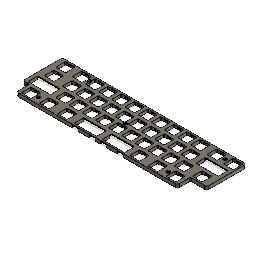
plate (Autodesk Fusion 360 design; units mm, degrees)
Autodesk Fusion 360 part; units mm, degrees
(part 1 of 9)
sketch "Sketch1" plane through (0, 0, 0) normal (0, 1, 0) x (1, 0, 0)
  line L0 (3, 0) -> (263.7, 0)
  line L1 (266.7, -3) -> (266.7, -73.2)
  line L2 (263.7, -76.2) -> (3, -76.2)
  line L3 (0, -73.2) -> (0, -3)
  arc A0 (3, 0) -> (0, -3) centre (3, -3) ccw
  arc A1 (0, -73.2) -> (3, -76.2) centre (3, -73.2) ccw
  arc A2 (266.7, -3) -> (263.7, 0) centre (263.7, -3) ccw
  arc A3 (263.7, -76.2) -> (266.7, -73.2) centre (263.7, -73.2) ccw
  point P0 (266.7, 0)
  point P1 (0, -76.2)
  dimension "d1" = 266.7
  dimension "d2" = 76.2
  dimension "d3" = 3
  constraint horizontal L0
  constraint vertical L1
  constraint horizontal L2
  constraint vertical L3
  constraint coincident origin L0
  constraint coincident origin L3
  constraint tangent L0 A0
  constraint tangent L3 A0
  constraint coincident P1 L2
  constraint coincident P1 L3
  constraint tangent L2 A1
  constraint tangent L3 A1
  constraint equal A0 A1
  constraint coincident P0 L0
  constraint coincident P0 L1
  constraint tangent L0 A2
  constraint tangent L1 A2
  constraint equal A0 A2
  constraint tangent L1 A3
  constraint tangent L2 A3
  constraint equal A0 A3
  measures "d1" distance of origin P0
  measures "d2" distance of origin P1
  measures "d3" radius of A0
extrude "Extrude1" add sketch "Sketch1" along normal blind 5.1
sketch "Sketch2" plane through (0, 5.1, 0) normal (0, 1, 0) x (-1, 0, 0)
  arc A0 (0, 73.2) -> (-3, 76.2) centre (-3, 73.2) ccw
  line L0 (-3, 76.2) -> (-263.7, 76.2)
  arc A1 (-263.7, 76.2) -> (-266.7, 73.2) centre (-263.7, 73.2) ccw
  line L1 (-266.7, 73.2) -> (-266.7, 3)
  arc A2 (-266.7, 3) -> (-263.7, 0) centre (-263.7, 3) ccw
  line L2 (-263.7, 0) -> (-3, 0)
  arc A3 (-3, 0) -> (0, 3) centre (-3, 3) ccw
  line L3 (0, 3) -> (0, 73.2)
  line L4 (0, 57.15) -> (-8.525, 57.15)
  line L5 (-9.525, 58.15) -> (-9.525, 76.2)
  line L6 (-9.525, 76.2) -> (0, 76.2)
  line L7 (0, 76.2) -> (0, 57.15)
  arc A4 (-9.525, 58.15) -> (-8.525, 57.15) centre (-8.525, 58.15) ccw
  line L8 (-266.7, 57.15) -> (-243.8875, 57.15)
  line L9 (-242.8875, 58.15) -> (-242.8875, 76.2)
  line L10 (-242.8875, 76.2) -> (-266.7, 76.2)
  line L11 (-266.7, 76.2) -> (-266.7, 57.15)
  arc A5 (-243.8875, 57.15) -> (-242.8875, 58.15) centre (-243.8875, 58.15) ccw
  point P0 (-9.525, 57.15)
  point P1 (-242.8875, 57.15)
  dimension "d6" = 19.05
  dimension "d7" = 9.525
  dimension "d8" = 1
  dimension "d9" = 19.05
  dimension "d10" = 23.8125
  dimension "d11" = 1
  constraint horizontal L4
  constraint vertical L5
  constraint horizontal L6
  constraint vertical L7
  constraint coincident L0 L5.end
  constraint coincident L3 L4.start
  constraint coincident P0 L4
  constraint coincident P0 L5
  constraint tangent L4 A4
  constraint tangent L5 A4
  constraint horizontal L8
  constraint vertical L9
  constraint horizontal L10
  constraint vertical L11
  constraint coincident L0 L9.end
  constraint coincident L1 L8.start
  constraint coincident P1 L8
  constraint coincident P1 L9
  constraint tangent L8 A5
  constraint tangent L9 A5
  measures "d6" distance of P0 L5.end
  measures "d7" distance of L4.start P0
  measures "d8" radius of A4
  measures "d9" distance of P1 L9.end
  measures "d10" distance of L8.start P1
  measures "d11" radius of A5
extrude "Extrude2" cut sketch "Sketch2" against normal blind 5.1 contours A0 L0 L3 L4 L5 L6 L7 A4 | L0 A1 L1 L8 L9 L10 L11 A5
fillet "Fillet1" radius 3 2 edges at (0, 2.55, 57.15) (9.525, 2.55, 76.2)
fillet "Fillet2" radius 3 2 edges at (242.8875, 2.55, 76.2) (266.7, 2.55, 57.15)
sketch "Sketch3" plane through (0, 5.1, 0) normal (0, 1, 0) x (-1, 0, 0)
  arc A0 (-263.7, 57.15) -> (-266.7, 54.15) centre (-263.7, 54.15) ccw
  line L0 (-266.7, 54.15) -> (-266.7, 3)
  arc A1 (-266.7, 3) -> (-263.7, 0) centre (-263.7, 3) ccw
  line L1 (-263.7, 0) -> (-3, 0)
  arc A2 (-3, 0) -> (0, 3) centre (-3, 3) ccw
  line L2 (0, 3) -> (0, 54.15)
  arc A3 (0, 54.15) -> (-3, 57.15) centre (-3, 54.15) ccw
  line L3 (-3, 57.15) -> (-8.525, 57.15)
  arc A4 (-9.525, 58.15) -> (-8.525, 57.15) centre (-8.525, 58.15) ccw
  line L4 (-9.525, 58.15) -> (-9.525, 73.2)
  arc A5 (-9.525, 73.2) -> (-12.525, 76.2) centre (-12.525, 73.2) ccw
  line L5 (-12.525, 76.2) -> (-239.8875, 76.2)
  arc A6 (-239.8875, 76.2) -> (-242.8875, 73.2) centre (-239.8875, 73.2) ccw
  line L6 (-242.8875, 73.2) -> (-242.8875, 58.15)
  arc A7 (-243.8875, 57.15) -> (-242.8875, 58.15) centre (-243.8875, 58.15) ccw
  line L7 (-243.8875, 57.15) -> (-263.7, 57.15)
  line L8 (-3.525, 2.525) -> (-15.525, 2.525)
  line L9 (-16.525, 3.525) -> (-16.525, 15.525)
  line L10 (-15.525, 16.525) -> (-3.525, 16.525)
  line L11 (-2.525, 15.525) -> (-2.525, 3.525)
  arc A8 (-3.525, 2.525) -> (-2.525, 3.525) centre (-3.525, 3.525) ccw
  arc A9 (-16.525, 3.525) -> (-15.525, 2.525) centre (-15.525, 3.525) ccw
  arc A10 (-15.525, 16.525) -> (-16.525, 15.525) centre (-15.525, 15.525) ccw
  arc A11 (-2.525, 15.525) -> (-3.525, 16.525) centre (-3.525, 15.525) ccw
  arc A12 (-45.1, 3.525) -> (-44.1, 2.525) centre (-44.1, 3.525) ccw
  line L12 (-32.1, 2.525) -> (-44.1, 2.525)
  arc A13 (-32.1, 2.525) -> (-31.1, 3.525) centre (-32.1, 3.525) ccw
  line L13 (-31.1, 15.525) -> (-31.1, 3.525)
  arc A14 (-31.1, 15.525) -> (-32.1, 16.525) centre (-32.1, 15.525) ccw
  line L14 (-44.1, 16.525) -> (-32.1, 16.525)
  line L15 (-45.1, 3.525) -> (-45.1, 15.525)
  arc A15 (-44.1, 16.525) -> (-45.1, 15.525) centre (-44.1, 15.525) ccw
  line L16 (-51.15, 2.525) -> (-63.15, 2.525)
  line L17 (-64.15, 3.525) -> (-64.15, 15.525)
  line L18 (-63.15, 16.525) -> (-51.15, 16.525)
  line L19 (-50.15, 15.525) -> (-50.15, 3.525)
  arc A16 (-64.15, 3.525) -> (-63.15, 2.525) centre (-63.15, 3.525) ccw
  arc A17 (-63.15, 16.525) -> (-64.15, 15.525) centre (-63.15, 15.525) ccw
  arc A18 (-51.15, 2.525) -> (-50.15, 3.525) centre (-51.15, 3.525) ccw
  arc A19 (-50.15, 15.525) -> (-51.15, 16.525) centre (-51.15, 15.525) ccw
  line L20 (-70.2, 2.525) -> (-82.2, 2.525)
  line L21 (-83.2, 3.525) -> (-83.2, 15.525)
  line L22 (-82.2, 16.525) -> (-70.2, 16.525)
  line L23 (-69.2, 15.525) -> (-69.2, 3.525)
  arc A20 (-83.2, 3.525) -> (-82.2, 2.525) centre (-82.2, 3.525) ccw
  arc A21 (-82.2, 16.525) -> (-83.2, 15.525) centre (-82.2, 15.525) ccw
  arc A22 (-70.2, 2.525) -> (-69.2, 3.525) centre (-70.2, 3.525) ccw
  arc A23 (-69.2, 15.525) -> (-70.2, 16.525) centre (-70.2, 15.525) ccw
  line L24 (-89.25, 2.525) -> (-101.25, 2.525)
  line L25 (-102.25, 3.525) -> (-102.25, 15.525)
  line L26 (-101.25, 16.525) -> (-89.25, 16.525)
  line L27 (-88.25, 15.525) -> (-88.25, 3.525)
  arc A24 (-102.25, 3.525) -> (-101.25, 2.525) centre (-101.25, 3.525) ccw
  arc A25 (-101.25, 16.525) -> (-102.25, 15.525) centre (-101.25, 15.525) ccw
  arc A26 (-89.25, 2.525) -> (-88.25, 3.525) centre (-89.25, 3.525) ccw
  arc A27 (-88.25, 15.525) -> (-89.25, 16.525) centre (-89.25, 15.525) ccw
  line L28 (-108.3, 2.525) -> (-120.3, 2.525)
  line L29 (-121.3, 3.525) -> (-121.3, 15.525)
  line L30 (-120.3, 16.525) -> (-108.3, 16.525)
  line L31 (-107.3, 15.525) -> (-107.3, 3.525)
  arc A28 (-121.3, 3.525) -> (-120.3, 2.525) centre (-120.3, 3.525) ccw
  arc A29 (-120.3, 16.525) -> (-121.3, 15.525) centre (-120.3, 15.525) ccw
  arc A30 (-108.3, 2.525) -> (-107.3, 3.525) centre (-108.3, 3.525) ccw
  arc A31 (-107.3, 15.525) -> (-108.3, 16.525) centre (-108.3, 15.525) ccw
  line L32 (-127.35, 2.525) -> (-139.35, 2.525)
  line L33 (-140.35, 3.525) -> (-140.35, 15.525)
  line L34 (-139.35, 16.525) -> (-127.35, 16.525)
  line L35 (-126.35, 15.525) -> (-126.35, 3.525)
  arc A32 (-140.35, 3.525) -> (-139.35, 2.525) centre (-139.35, 3.525) ccw
  arc A33 (-139.35, 16.525) -> (-140.35, 15.525) centre (-139.35, 15.525) ccw
  arc A34 (-127.35, 2.525) -> (-126.35, 3.525) centre (-127.35, 3.525) ccw
  arc A35 (-126.35, 15.525) -> (-127.35, 16.525) centre (-127.35, 15.525) ccw
  line L36 (-146.4, 2.525) -> (-158.4, 2.525)
  line L37 (-159.4, 3.525) -> (-159.4, 15.525)
  line L38 (-158.4, 16.525) -> (-146.4, 16.525)
  line L39 (-145.4, 15.525) -> (-145.4, 3.525)
  arc A36 (-159.4, 3.525) -> (-158.4, 2.525) centre (-158.4, 3.525) ccw
  arc A37 (-158.4, 16.525) -> (-159.4, 15.525) centre (-158.4, 15.525) ccw
  arc A38 (-146.4, 2.525) -> (-145.4, 3.525) centre (-146.4, 3.525) ccw
  arc A39 (-145.4, 15.525) -> (-146.4, 16.525) centre (-146.4, 15.525) ccw
  line L40 (-165.45, 2.525) -> (-177.45, 2.525)
  line L41 (-178.45, 3.525) -> (-178.45, 15.525)
  line L42 (-177.45, 16.525) -> (-165.45, 16.525)
  line L43 (-164.45, 15.525) -> (-164.45, 3.525)
  arc A40 (-178.45, 3.525) -> (-177.45, 2.525) centre (-177.45, 3.525) ccw
  arc A41 (-177.45, 16.525) -> (-178.45, 15.525) centre (-177.45, 15.525) ccw
  arc A42 (-165.45, 2.525) -> (-164.45, 3.525) centre (-165.45, 3.525) ccw
  arc A43 (-164.45, 15.525) -> (-165.45, 16.525) centre (-165.45, 15.525) ccw
  line L44 (-184.5, 2.525) -> (-196.5, 2.525)
  line L45 (-197.5, 3.525) -> (-197.5, 15.525)
  line L46 (-196.5, 16.525) -> (-184.5, 16.525)
  line L47 (-183.5, 15.525) -> (-183.5, 3.525)
  arc A44 (-197.5, 3.525) -> (-196.5, 2.525) centre (-196.5, 3.525) ccw
  arc A45 (-196.5, 16.525) -> (-197.5, 15.525) centre (-196.5, 15.525) ccw
  arc A46 (-184.5, 2.525) -> (-183.5, 3.525) centre (-184.5, 3.525) ccw
  arc A47 (-183.5, 15.525) -> (-184.5, 16.525) centre (-184.5, 15.525) ccw
  line L48 (-203.55, 2.525) -> (-215.55, 2.525)
  line L49 (-216.55, 3.525) -> (-216.55, 15.525)
  line L50 (-215.55, 16.525) -> (-203.55, 16.525)
  line L51 (-202.55, 15.525) -> (-202.55, 3.525)
  arc A48 (-216.55, 3.525) -> (-215.55, 2.525) centre (-215.55, 3.525) ccw
  arc A49 (-215.55, 16.525) -> (-216.55, 15.525) centre (-215.55, 15.525) ccw
  arc A50 (-203.55, 2.525) -> (-202.55, 3.525) centre (-203.55, 3.525) ccw
  arc A51 (-202.55, 15.525) -> (-203.55, 16.525) centre (-203.55, 15.525) ccw
  line L52 (-227.3625, 2.525) -> (-239.3625, 2.525)
  line L53 (-240.3625, 3.525) -> (-240.3625, 15.525)
  line L54 (-239.3625, 16.525) -> (-227.3625, 16.525)
  line L55 (-226.3625, 15.525) -> (-226.3625, 3.525)
  arc A52 (-240.3625, 3.525) -> (-239.3625, 2.525) centre (-239.3625, 3.525) ccw
  arc A53 (-239.3625, 16.525) -> (-240.3625, 15.525) centre (-239.3625, 15.525) ccw
  arc A54 (-227.3625, 2.525) -> (-226.3625, 3.525) centre (-227.3625, 3.525) ccw
  arc A55 (-226.3625, 15.525) -> (-227.3625, 16.525) centre (-227.3625, 15.525) ccw
  line L56 (-251.175, 2.525) -> (-263.175, 2.525)
  line L57 (-264.175, 3.525) -> (-264.175, 15.525)
  line L58 (-263.175, 16.525) -> (-251.175, 16.525)
  line L59 (-250.175, 15.525) -> (-250.175, 3.525)
  arc A56 (-264.175, 3.525) -> (-263.175, 2.525) centre (-263.175, 3.525) ccw
  arc A57 (-263.175, 16.525) -> (-264.175, 15.525) centre (-263.175, 15.525) ccw
  arc A58 (-251.175, 2.525) -> (-250.175, 3.525) centre (-251.175, 3.525) ccw
  arc A59 (-250.175, 15.525) -> (-251.175, 16.525) centre (-251.175, 15.525) ccw
  line L60 (-10.6687, 21.575) -> (-22.6688, 21.575)
  line L61 (-23.6688, 22.575) -> (-23.6688, 34.575)
  line L62 (-22.6688, 35.575) -> (-10.6688, 35.575)
  line L63 (-9.6688, 34.575) -> (-9.6688, 22.575)
  arc A60 (-23.6688, 22.575) -> (-22.6688, 21.575) centre (-22.6688, 22.575) ccw
  arc A61 (-22.6687, 35.575) -> (-23.6687, 34.575) centre (-22.6687, 34.575) ccw
  arc A62 (-10.6687, 21.575) -> (-9.6687, 22.575) centre (-10.6687, 22.575) ccw
  arc A63 (-9.6688, 34.575) -> (-10.6688, 35.575) centre (-10.6688, 34.575) ccw
  line L64 (-36.8625, 21.575) -> (-48.8625, 21.575)
  line L65 (-49.8625, 22.575) -> (-49.8625, 34.575)
  line L66 (-48.8625, 35.575) -> (-36.8625, 35.575)
  line L67 (-35.8625, 34.575) -> (-35.8625, 22.575)
  arc A64 (-49.8625, 22.575) -> (-48.8625, 21.575) centre (-48.8625, 22.575) ccw
  arc A65 (-48.8625, 35.575) -> (-49.8625, 34.575) centre (-48.8625, 34.575) ccw
  arc A66 (-36.8625, 21.575) -> (-35.8625, 22.575) centre (-36.8625, 22.575) ccw
  arc A67 (-35.8625, 34.575) -> (-36.8625, 35.575) centre (-36.8625, 34.575) ccw
  line L68 (-55.9125, 21.575) -> (-67.9125, 21.575)
  line L69 (-68.9125, 22.575) -> (-68.9125, 34.575)
  line L70 (-67.9125, 35.575) -> (-55.9125, 35.575)
  line L71 (-54.9125, 34.575) -> (-54.9125, 22.575)
  arc A68 (-68.9125, 22.575) -> (-67.9125, 21.575) centre (-67.9125, 22.575) ccw
  arc A69 (-67.9125, 35.575) -> (-68.9125, 34.575) centre (-67.9125, 34.575) ccw
  arc A70 (-55.9125, 21.575) -> (-54.9125, 22.575) centre (-55.9125, 22.575) ccw
  arc A71 (-54.9125, 34.575) -> (-55.9125, 35.575) centre (-55.9125, 34.575) ccw
  line L72 (-74.9625, 21.575) -> (-86.9625, 21.575)
  line L73 (-87.9625, 22.575) -> (-87.9625, 34.575)
  line L74 (-86.9625, 35.575) -> (-74.9625, 35.575)
  line L75 (-73.9625, 34.575) -> (-73.9625, 22.575)
  arc A72 (-87.9625, 22.575) -> (-86.9625, 21.575) centre (-86.9625, 22.575) ccw
  arc A73 (-86.9625, 35.575) -> (-87.9625, 34.575) centre (-86.9625, 34.575) ccw
  arc A74 (-74.9625, 21.575) -> (-73.9625, 22.575) centre (-74.9625, 22.575) ccw
  arc A75 (-73.9625, 34.575) -> (-74.9625, 35.575) centre (-74.9625, 34.575) ccw
  line L76 (-94.0125, 21.575) -> (-106.0125, 21.575)
  line L77 (-107.0125, 22.575) -> (-107.0125, 34.575)
  line L78 (-106.0125, 35.575) -> (-94.0125, 35.575)
  line L79 (-93.0125, 34.575) -> (-93.0125, 22.575)
  arc A76 (-107.0125, 22.575) -> (-106.0125, 21.575) centre (-106.0125, 22.575) ccw
  arc A77 (-106.0125, 35.575) -> (-107.0125, 34.575) centre (-106.0125, 34.575) ccw
  arc A78 (-94.0125, 21.575) -> (-93.0125, 22.575) centre (-94.0125, 22.575) ccw
  arc A79 (-93.0125, 34.575) -> (-94.0125, 35.575) centre (-94.0125, 34.575) ccw
  line L80 (-113.0625, 21.575) -> (-125.0625, 21.575)
  line L81 (-126.0625, 22.575) -> (-126.0625, 34.575)
  line L82 (-125.0625, 35.575) -> (-113.0625, 35.575)
  line L83 (-112.0625, 34.575) -> (-112.0625, 22.575)
  arc A80 (-126.0625, 22.575) -> (-125.0625, 21.575) centre (-125.0625, 22.575) ccw
  arc A81 (-125.0625, 35.575) -> (-126.0625, 34.575) centre (-125.0625, 34.575) ccw
  arc A82 (-113.0625, 21.575) -> (-112.0625, 22.575) centre (-113.0625, 22.575) ccw
  arc A83 (-112.0625, 34.575) -> (-113.0625, 35.575) centre (-113.0625, 34.575) ccw
  line L84 (-132.1125, 21.575) -> (-144.1125, 21.575)
  line L85 (-145.1125, 22.575) -> (-145.1125, 34.575)
  line L86 (-144.1125, 35.575) -> (-132.1125, 35.575)
  line L87 (-131.1125, 34.575) -> (-131.1125, 22.575)
  arc A84 (-145.1125, 22.575) -> (-144.1125, 21.575) centre (-144.1125, 22.575) ccw
  arc A85 (-144.1125, 35.575) -> (-145.1125, 34.575) centre (-144.1125, 34.575) ccw
  arc A86 (-132.1125, 21.575) -> (-131.1125, 22.575) centre (-132.1125, 22.575) ccw
  arc A87 (-131.1125, 34.575) -> (-132.1125, 35.575) centre (-132.1125, 34.575) ccw
  line L88 (-151.1625, 21.575) -> (-163.1625, 21.575)
  line L89 (-164.1625, 22.575) -> (-164.1625, 34.575)
  line L90 (-163.1625, 35.575) -> (-151.1625, 35.575)
  line L91 (-150.1625, 34.575) -> (-150.1625, 22.575)
  arc A88 (-164.1625, 22.575) -> (-163.1625, 21.575) centre (-163.1625, 22.575) ccw
  arc A89 (-163.1625, 35.575) -> (-164.1625, 34.575) centre (-163.1625, 34.575) ccw
  arc A90 (-151.1625, 21.575) -> (-150.1625, 22.575) centre (-151.1625, 22.575) ccw
  arc A91 (-150.1625, 34.575) -> (-151.1625, 35.575) centre (-151.1625, 34.575) ccw
  line L92 (-170.2125, 21.575) -> (-182.2125, 21.575)
  line L93 (-183.2125, 22.575) -> (-183.2125, 34.575)
  line L94 (-182.2125, 35.575) -> (-170.2125, 35.575)
  line L95 (-169.2125, 34.575) -> (-169.2125, 22.575)
  arc A92 (-183.2125, 22.575) -> (-182.2125, 21.575) centre (-182.2125, 22.575) ccw
  arc A93 (-182.2125, 35.575) -> (-183.2125, 34.575) centre (-182.2125, 34.575) ccw
  arc A94 (-170.2125, 21.575) -> (-169.2125, 22.575) centre (-170.2125, 22.575) ccw
  arc A95 (-169.2125, 34.575) -> (-170.2125, 35.575) centre (-170.2125, 34.575) ccw
  line L96 (-189.2625, 21.575) -> (-201.2625, 21.575)
  line L97 (-202.2625, 22.575) -> (-202.2625, 34.575)
  line L98 (-201.2625, 35.575) -> (-189.2625, 35.575)
  line L99 (-188.2625, 34.575) -> (-188.2625, 22.575)
  arc A96 (-202.2625, 22.575) -> (-201.2625, 21.575) centre (-201.2625, 22.575) ccw
  arc A97 (-201.2625, 35.575) -> (-202.2625, 34.575) centre (-201.2625, 34.575) ccw
  arc A98 (-189.2625, 21.575) -> (-188.2625, 22.575) centre (-189.2625, 22.575) ccw
  arc A99 (-188.2625, 34.575) -> (-189.2625, 35.575) centre (-189.2625, 34.575) ccw
  line L100 (-208.3125, 21.575) -> (-220.3125, 21.575)
  line L101 (-221.3125, 22.575) -> (-221.3125, 34.575)
  line L102 (-220.3125, 35.575) -> (-208.3125, 35.575)
  line L103 (-207.3125, 34.575) -> (-207.3125, 22.575)
  arc A100 (-221.3125, 22.575) -> (-220.3125, 21.575) centre (-220.3125, 22.575) ccw
  arc A101 (-220.3125, 35.575) -> (-221.3125, 34.575) centre (-220.3125, 34.575) ccw
  arc A102 (-208.3125, 21.575) -> (-207.3125, 22.575) centre (-208.3125, 22.575) ccw
  arc A103 (-207.3125, 34.575) -> (-208.3125, 35.575) centre (-208.3125, 34.575) ccw
  line L104 (-239.2688, 21.575) -> (-251.2688, 21.575)
  line L105 (-252.2688, 22.575) -> (-252.2688, 34.575)
  line L106 (-251.2688, 35.575) -> (-239.2688, 35.575)
  line L107 (-238.2688, 34.575) -> (-238.2688, 22.575)
  arc A104 (-252.2688, 22.575) -> (-251.2688, 21.575) centre (-251.2688, 22.575) ccw
  arc A105 (-251.2688, 35.575) -> (-252.2687, 34.575) centre (-251.2687, 34.575) ccw
  arc A106 (-239.2688, 21.575) -> (-238.2688, 22.575) centre (-239.2688, 22.575) ccw
  arc A107 (-238.2688, 34.575) -> (-239.2688, 35.575) centre (-239.2688, 34.575) ccw
  line L108 (-15.4313, 40.625) -> (-27.4313, 40.625)
  line L109 (-28.4313, 41.625) -> (-28.4313, 53.625)
  line L110 (-27.4313, 54.625) -> (-15.4313, 54.625)
  line L111 (-14.4313, 53.625) -> (-14.4313, 41.625)
  arc A108 (-28.4313, 41.625) -> (-27.4313, 40.625) centre (-27.4313, 41.625) ccw
  arc A109 (-27.4313, 54.625) -> (-28.4313, 53.625) centre (-27.4312, 53.625) ccw
  arc A110 (-15.4313, 40.625) -> (-14.4313, 41.625) centre (-15.4313, 41.625) ccw
  arc A111 (-14.4313, 53.625) -> (-15.4313, 54.625) centre (-15.4313, 53.625) ccw
  line L112 (-46.3875, 40.625) -> (-58.3875, 40.625)
  line L113 (-59.3875, 41.625) -> (-59.3875, 53.625)
  line L114 (-58.3875, 54.625) -> (-46.3875, 54.625)
  line L115 (-45.3875, 53.625) -> (-45.3875, 41.625)
  arc A112 (-59.3875, 41.625) -> (-58.3875, 40.625) centre (-58.3875, 41.625) ccw
  arc A113 (-58.3875, 54.625) -> (-59.3875, 53.625) centre (-58.3875, 53.625) ccw
  arc A114 (-46.3875, 40.625) -> (-45.3875, 41.625) centre (-46.3875, 41.625) ccw
  arc A115 (-45.3875, 53.625) -> (-46.3875, 54.625) centre (-46.3875, 53.625) ccw
  line L116 (-65.4375, 40.625) -> (-77.4375, 40.625)
  line L117 (-78.4375, 41.625) -> (-78.4375, 53.625)
  line L118 (-77.4375, 54.625) -> (-65.4375, 54.625)
  line L119 (-64.4375, 53.625) -> (-64.4375, 41.625)
  arc A116 (-78.4375, 41.625) -> (-77.4375, 40.625) centre (-77.4375, 41.625) ccw
  arc A117 (-77.4375, 54.625) -> (-78.4375, 53.625) centre (-77.4375, 53.625) ccw
  arc A118 (-65.4375, 40.625) -> (-64.4375, 41.625) centre (-65.4375, 41.625) ccw
  arc A119 (-64.4375, 53.625) -> (-65.4375, 54.625) centre (-65.4375, 53.625) ccw
  line L120 (-84.4875, 40.625) -> (-96.4875, 40.625)
  line L121 (-97.4875, 41.625) -> (-97.4875, 53.625)
  line L122 (-96.4875, 54.625) -> (-84.4875, 54.625)
  line L123 (-83.4875, 53.625) -> (-83.4875, 41.625)
  arc A120 (-97.4875, 41.625) -> (-96.4875, 40.625) centre (-96.4875, 41.625) ccw
  arc A121 (-96.4875, 54.625) -> (-97.4875, 53.625) centre (-96.4875, 53.625) ccw
  arc A122 (-84.4875, 40.625) -> (-83.4875, 41.625) centre (-84.4875, 41.625) ccw
  arc A123 (-83.4875, 53.625) -> (-84.4875, 54.625) centre (-84.4875, 53.625) ccw
  line L124 (-103.5375, 40.625) -> (-115.5375, 40.625)
  line L125 (-116.5375, 41.625) -> (-116.5375, 53.625)
  line L126 (-115.5375, 54.625) -> (-103.5375, 54.625)
  line L127 (-102.5375, 53.625) -> (-102.5375, 41.625)
  arc A124 (-116.5375, 41.625) -> (-115.5375, 40.625) centre (-115.5375, 41.625) ccw
  arc A125 (-115.5375, 54.625) -> (-116.5375, 53.625) centre (-115.5375, 53.625) ccw
  arc A126 (-103.5375, 40.625) -> (-102.5375, 41.625) centre (-103.5375, 41.625) ccw
  arc A127 (-102.5375, 53.625) -> (-103.5375, 54.625) centre (-103.5375, 53.625) ccw
  line L128 (-122.5875, 40.625) -> (-134.5875, 40.625)
  line L129 (-135.5875, 41.625) -> (-135.5875, 53.625)
  line L130 (-134.5875, 54.625) -> (-122.5875, 54.625)
  line L131 (-121.5875, 53.625) -> (-121.5875, 41.625)
  arc A128 (-135.5875, 41.625) -> (-134.5875, 40.625) centre (-134.5875, 41.625) ccw
  arc A129 (-134.5875, 54.625) -> (-135.5875, 53.625) centre (-134.5875, 53.625) ccw
  arc A130 (-122.5875, 40.625) -> (-121.5875, 41.625) centre (-122.5875, 41.625) ccw
  arc A131 (-121.5875, 53.625) -> (-122.5875, 54.625) centre (-122.5875, 53.625) ccw
  line L132 (-141.6375, 40.625) -> (-153.6375, 40.625)
  line L133 (-154.6375, 41.625) -> (-154.6375, 53.625)
  line L134 (-153.6375, 54.625) -> (-141.6375, 54.625)
  line L135 (-140.6375, 53.625) -> (-140.6375, 41.625)
  arc A132 (-154.6375, 41.625) -> (-153.6375, 40.625) centre (-153.6375, 41.625) ccw
  arc A133 (-153.6375, 54.625) -> (-154.6375, 53.625) centre (-153.6375, 53.625) ccw
  arc A134 (-141.6375, 40.625) -> (-140.6375, 41.625) centre (-141.6375, 41.625) ccw
  arc A135 (-140.6375, 53.625) -> (-141.6375, 54.625) centre (-141.6375, 53.625) ccw
  line L136 (-160.6875, 40.625) -> (-172.6875, 40.625)
  line L137 (-173.6875, 41.625) -> (-173.6875, 53.625)
  line L138 (-172.6875, 54.625) -> (-160.6875, 54.625)
  line L139 (-159.6875, 53.625) -> (-159.6875, 41.625)
  arc A136 (-173.6875, 41.625) -> (-172.6875, 40.625) centre (-172.6875, 41.625) ccw
  arc A137 (-172.6875, 54.625) -> (-173.6875, 53.625) centre (-172.6875, 53.625) ccw
  arc A138 (-160.6875, 40.625) -> (-159.6875, 41.625) centre (-160.6875, 41.625) ccw
  arc A139 (-159.6875, 53.625) -> (-160.6875, 54.625) centre (-160.6875, 53.625) ccw
  line L140 (-179.7375, 40.625) -> (-191.7375, 40.625)
  line L141 (-192.7375, 41.625) -> (-192.7375, 53.625)
  line L142 (-191.7375, 54.625) -> (-179.7375, 54.625)
  line L143 (-178.7375, 53.625) -> (-178.7375, 41.625)
  arc A140 (-192.7375, 41.625) -> (-191.7375, 40.625) centre (-191.7375, 41.625) ccw
  arc A141 (-191.7375, 54.625) -> (-192.7375, 53.625) centre (-191.7375, 53.625) ccw
  arc A142 (-179.7375, 40.625) -> (-178.7375, 41.625) centre (-179.7375, 41.625) ccw
  arc A143 (-178.7375, 53.625) -> (-179.7375, 54.625) centre (-179.7375, 53.625) ccw
  line L144 (-198.7875, 40.625) -> (-210.7875, 40.625)
  line L145 (-211.7875, 41.625) -> (-211.7875, 53.625)
  line L146 (-210.7875, 54.625) -> (-198.7875, 54.625)
  line L147 (-197.7875, 53.625) -> (-197.7875, 41.625)
  arc A144 (-211.7875, 41.625) -> (-210.7875, 40.625) centre (-210.7875, 41.625) ccw
  arc A145 (-210.7875, 54.625) -> (-211.7875, 53.625) centre (-210.7875, 53.625) ccw
  arc A146 (-198.7875, 40.625) -> (-197.7875, 41.625) centre (-198.7875, 41.625) ccw
  arc A147 (-197.7875, 53.625) -> (-198.7875, 54.625) centre (-198.7875, 53.625) ccw
  line L148 (-217.8375, 40.625) -> (-229.8375, 40.625)
  line L149 (-230.8375, 41.625) -> (-230.8375, 53.625)
  line L150 (-229.8375, 54.625) -> (-217.8375, 54.625)
  line L151 (-216.8375, 53.625) -> (-216.8375, 41.625)
  arc A148 (-230.8375, 41.625) -> (-229.8375, 40.625) centre (-229.8375, 41.625) ccw
  arc A149 (-229.8375, 54.625) -> (-230.8375, 53.625) centre (-229.8375, 53.625) ccw
  arc A150 (-217.8375, 40.625) -> (-216.8375, 41.625) centre (-217.8375, 41.625) ccw
  arc A151 (-216.8375, 53.625) -> (-217.8375, 54.625) centre (-217.8375, 53.625) ccw
  line L152 (-244.0312, 40.625) -> (-256.0312, 40.625)
  line L153 (-257.0312, 41.625) -> (-257.0312, 53.625)
  line L154 (-256.0312, 54.625) -> (-244.0312, 54.625)
  line L155 (-243.0312, 53.625) -> (-243.0312, 41.625)
  arc A152 (-257.0312, 41.625) -> (-256.0312, 40.625) centre (-256.0312, 41.625) ccw
  arc A153 (-256.0312, 54.625) -> (-257.0312, 53.625) centre (-256.0312, 53.625) ccw
  arc A154 (-244.0312, 40.625) -> (-243.0312, 41.625) centre (-244.0312, 41.625) ccw
  arc A155 (-243.0313, 53.625) -> (-244.0312, 54.625) centre (-244.0312, 53.625) ccw
  line L156 (-15.4313, 59.675) -> (-27.4313, 59.675)
  line L157 (-28.4313, 60.675) -> (-28.4313, 72.675)
  line L158 (-27.4313, 73.675) -> (-15.4313, 73.675)
  line L159 (-14.4313, 72.675) -> (-14.4313, 60.675)
  arc A156 (-28.4313, 60.675) -> (-27.4313, 59.675) centre (-27.4313, 60.675) ccw
  arc A157 (-27.4313, 73.675) -> (-28.4312, 72.675) centre (-27.4312, 72.675) ccw
  arc A158 (-15.4313, 59.675) -> (-14.4313, 60.675) centre (-15.4313, 60.675) ccw
  arc A159 (-14.4313, 72.675) -> (-15.4313, 73.675) centre (-15.4313, 72.675) ccw
  line L160 (-41.625, 59.675) -> (-53.625, 59.675)
  line L161 (-54.625, 60.675) -> (-54.625, 72.675)
  line L162 (-53.625, 73.675) -> (-41.625, 73.675)
  line L163 (-40.625, 72.675) -> (-40.625, 60.675)
  arc A160 (-54.625, 60.675) -> (-53.625, 59.675) centre (-53.625, 60.675) ccw
  arc A161 (-53.625, 73.675) -> (-54.625, 72.675) centre (-53.625, 72.675) ccw
  arc A162 (-41.625, 59.675) -> (-40.625, 60.675) centre (-41.625, 60.675) ccw
  arc A163 (-40.625, 72.675) -> (-41.625, 73.675) centre (-41.625, 72.675) ccw
  line L164 (-67.8188, 59.675) -> (-79.8188, 59.675)
  line L165 (-80.8187, 60.675) -> (-80.8187, 72.675)
  line L166 (-79.8188, 73.675) -> (-67.8188, 73.675)
  line L167 (-66.8188, 72.675) -> (-66.8188, 60.675)
  arc A164 (-80.8188, 60.675) -> (-79.8188, 59.675) centre (-79.8188, 60.675) ccw
  arc A165 (-79.8188, 73.675) -> (-80.8188, 72.675) centre (-79.8188, 72.675) ccw
  arc A166 (-67.8188, 59.675) -> (-66.8188, 60.675) centre (-67.8188, 60.675) ccw
  arc A167 (-66.8188, 72.675) -> (-67.8188, 73.675) centre (-67.8188, 72.675) ccw
  line L168 (-101.1563, 59.675) -> (-113.1562, 59.675)
  line L169 (-114.1562, 60.675) -> (-114.1562, 72.675)
  line L170 (-113.1562, 73.675) -> (-101.1562, 73.675)
  line L171 (-100.1562, 72.675) -> (-100.1562, 60.675)
  arc A168 (-114.1562, 60.675) -> (-113.1562, 59.675) centre (-113.1562, 60.675) ccw
  arc A169 (-113.1562, 73.675) -> (-114.1562, 72.675) centre (-113.1562, 72.675) ccw
  arc A170 (-101.1563, 59.675) -> (-100.1562, 60.675) centre (-101.1562, 60.675) ccw
  arc A171 (-100.1562, 72.675) -> (-101.1563, 73.675) centre (-101.1563, 72.675) ccw
  line L172 (-141.6375, 59.675) -> (-153.6375, 59.675)
  line L173 (-154.6375, 60.675) -> (-154.6375, 72.675)
  line L174 (-153.6375, 73.675) -> (-141.6375, 73.675)
  line L175 (-140.6375, 72.675) -> (-140.6375, 60.675)
  arc A172 (-154.6375, 60.675) -> (-153.6375, 59.675) centre (-153.6375, 60.675) ccw
  arc A173 (-153.6375, 73.675) -> (-154.6375, 72.675) centre (-153.6375, 72.675) ccw
  arc A174 (-141.6375, 59.675) -> (-140.6375, 60.675) centre (-141.6375, 60.675) ccw
  arc A175 (-140.6375, 72.675) -> (-141.6375, 73.675) centre (-141.6375, 72.675) ccw
  line L176 (-172.5938, 59.675) -> (-184.5938, 59.675)
  line L177 (-185.5938, 60.675) -> (-185.5938, 72.675)
  line L178 (-184.5938, 73.675) -> (-172.5937, 73.675)
  line L179 (-171.5938, 72.675) -> (-171.5938, 60.675)
  arc A176 (-185.5937, 60.675) -> (-184.5938, 59.675) centre (-184.5938, 60.675) ccw
  arc A177 (-184.5938, 73.675) -> (-185.5937, 72.675) centre (-184.5937, 72.675) ccw
  arc A178 (-172.5938, 59.675) -> (-171.5938, 60.675) centre (-172.5938, 60.675) ccw
  arc A179 (-171.5938, 72.675) -> (-172.5938, 73.675) centre (-172.5938, 72.675) ccw
  line L180 (-198.7875, 59.675) -> (-210.7875, 59.675)
  line L181 (-211.7875, 60.675) -> (-211.7875, 72.675)
  line L182 (-210.7875, 73.675) -> (-198.7875, 73.675)
  line L183 (-197.7875, 72.675) -> (-197.7875, 60.675)
  arc A180 (-211.7875, 60.675) -> (-210.7875, 59.675) centre (-210.7875, 60.675) ccw
  arc A181 (-210.7875, 73.675) -> (-211.7875, 72.675) centre (-210.7875, 72.675) ccw
  arc A182 (-198.7875, 59.675) -> (-197.7875, 60.675) centre (-198.7875, 60.675) ccw
  arc A183 (-197.7875, 72.675) -> (-198.7875, 73.675) centre (-198.7875, 72.675) ccw
  line L184 (-224.9813, 59.675) -> (-236.9813, 59.675)
  line L185 (-237.9813, 60.675) -> (-237.9813, 72.675)
  line L186 (-236.9813, 73.675) -> (-224.9813, 73.675)
  line L187 (-223.9813, 72.675) -> (-223.9813, 60.675)
  arc A184 (-237.9813, 60.675) -> (-236.9813, 59.675) centre (-236.9813, 60.675) ccw
  arc A185 (-236.9813, 73.675) -> (-237.9813, 72.675) centre (-236.9813, 72.675) ccw
  arc A186 (-224.9813, 59.675) -> (-223.9813, 60.675) centre (-224.9813, 60.675) ccw
  arc A187 (-223.9813, 72.675) -> (-224.9813, 73.675) centre (-224.9813, 72.675) ccw
  line L188 (-8.2875, 2.525) -> (-20.2875, 2.525)
  line L189 (-21.2875, 3.525) -> (-21.2875, 15.525)
  line L190 (-20.2875, 16.525) -> (-8.2875, 16.525)
  line L191 (-7.2875, 15.525) -> (-7.2875, 3.525)
  arc A188 (-21.2875, 3.525) -> (-20.2875, 2.525) centre (-20.2875, 3.525) ccw
  arc A189 (-20.2875, 16.525) -> (-21.2875, 15.525) centre (-20.2875, 15.525) ccw
  arc A190 (-8.2875, 2.525) -> (-7.2875, 3.525) centre (-8.2875, 3.525) ccw
  arc A191 (-7.2875, 15.525) -> (-8.2875, 16.525) centre (-8.2875, 15.525) ccw
  point P0 (-9.525, 9.525)
  point P1 (-2.525, 2.525)
  point P2 (-16.525, 2.525)
  point P3 (-2.525, 16.525)
  point P4 (-14.2875, 9.525)
  dimension "d16" = 9.525
  dimension "d17" = 9.525
  dimension "d18" = 14
  dimension "d19" = 14
  dimension "d20" = 7
  dimension "d21" = 7
  dimension "d22" = 1
  dimension "d23" = 4.7625
  dimension "d24" = 1
  dimension "d25" = 1
  dimension "d26" = 1
  dimension "d27" = 1
  dimension "d28" = 1
  dimension "d29" = 1
  dimension "d30" = 1
  dimension "d31" = 1
  dimension "d32" = 1
  dimension "d33" = 1
  dimension "d34" = 1
  dimension "d35" = 1
  dimension "d36" = 1
  dimension "d37" = 1
  dimension "d38" = 1
  dimension "d39" = 1
  dimension "d40" = 1
  dimension "d41" = 1
  dimension "d42" = 1
  dimension "d43" = 1
  dimension "d44" = 1
  dimension "d45" = 1
  dimension "d46" = 1
  dimension "d47" = 1
  dimension "d48" = 1
  dimension "d49" = 1
  dimension "d50" = 1
  dimension "d51" = 1
  dimension "d52" = 1
  dimension "d53" = 1
  dimension "d54" = 1
  dimension "d55" = 1
  dimension "d56" = 1
  dimension "d57" = 1
  dimension "d58" = 1
  dimension "d59" = 1
  dimension "d60" = 1
  dimension "d61" = 1
  dimension "d62" = 1
  dimension "d63" = 1
  dimension "d64" = 1
  dimension "d65" = 1
  dimension "d66" = 1
  dimension "d67" = 1
  dimension "d68" = 1
  constraint horizontal L8
  constraint vertical L9
  constraint horizontal L10
  constraint vertical L11
  constraint coincident P1 L8
  constraint coincident P1 L11
  constraint tangent L8 A8
  constraint tangent L11 A8
  constraint coincident P2 L8
  constraint coincident P2 L9
  constraint tangent L8 A9
  constraint tangent L9 A9
  constraint equal A8 A9
  constraint tangent L9 A10
  constraint tangent L10 A10
  constraint equal A8 A10
  constraint coincident P3 L10
  constraint coincident P3 L11
  constraint tangent L10 A11
  constraint tangent L11 A11
  constraint equal A8 A11
  constraint horizontal L12
  constraint vertical L15
  constraint horizontal L14
  constraint vertical L13
  constraint tangent L12 A13
  constraint tangent A13 L13
  constraint tangent A12 L12
  constraint tangent A12 L15
  constraint equal A12 A13
  constraint tangent L15 A15
  constraint tangent L14 A15
  constraint equal A13 A15
  constraint tangent A14 L14
  constraint tangent L13 A14
  constraint equal A13 A14
  constraint horizontal L16
  constraint vertical L17
  constraint horizontal L18
  constraint vertical L19
  constraint tangent L16 A18
  constraint tangent L19 A18
  constraint tangent L16 A16
  constraint tangent L17 A16
  constraint equal A16 A18
  constraint tangent L17 A17
  constraint tangent L18 A17
  constraint equal A17 A18
  constraint tangent L18 A19
  constraint tangent L19 A19
  constraint equal A18 A19
  constraint horizontal L20
  constraint vertical L21
  constraint horizontal L22
  constraint vertical L23
  constraint tangent L20 A22
  constraint tangent L23 A22
  constraint tangent L20 A20
  constraint tangent L21 A20
  constraint equal A20 A22
  constraint tangent L21 A21
  constraint tangent L22 A21
  constraint equal A21 A22
  constraint tangent L22 A23
  constraint tangent L23 A23
  constraint equal A22 A23
  constraint horizontal L24
  constraint vertical L25
  constraint horizontal L26
  constraint vertical L27
  constraint tangent L24 A26
  constraint tangent L27 A26
  constraint tangent L24 A24
  constraint tangent L25 A24
  constraint equal A24 A26
  constraint tangent L25 A25
  constraint tangent L26 A25
  constraint equal A25 A26
  constraint tangent L26 A27
  constraint tangent L27 A27
  constraint equal A26 A27
  constraint horizontal L28
  constraint vertical L29
  constraint horizontal L30
  constraint vertical L31
  constraint tangent L28 A30
  constraint tangent L31 A30
  constraint tangent L28 A28
  constraint tangent L29 A28
  constraint equal A28 A30
  constraint tangent L29 A29
  constraint tangent L30 A29
  constraint equal A29 A30
  constraint tangent L30 A31
  constraint tangent L31 A31
  constraint equal A30 A31
  constraint horizontal L32
  constraint vertical L33
  constraint horizontal L34
  constraint vertical L35
  constraint tangent L32 A34
  constraint tangent L35 A34
  constraint tangent L32 A32
  constraint tangent L33 A32
  constraint equal A32 A34
  constraint tangent L33 A33
  constraint tangent L34 A33
  constraint equal A33 A34
  constraint tangent L34 A35
  constraint tangent L35 A35
  constraint equal A34 A35
  constraint horizontal L36
  constraint vertical L37
  constraint horizontal L38
  constraint vertical L39
  constraint tangent L36 A38
  constraint tangent L39 A38
  constraint tangent L36 A36
  constraint tangent L37 A36
  constraint equal A36 A38
  constraint tangent L37 A37
  constraint tangent L38 A37
  constraint equal A37 A38
  constraint tangent L38 A39
  constraint tangent L39 A39
  constraint equal A38 A39
  constraint horizontal L40
  constraint vertical L41
  constraint horizontal L42
  constraint vertical L43
  constraint tangent L40 A42
  constraint tangent L43 A42
  constraint tangent L40 A40
  constraint tangent L41 A40
  constraint equal A40 A42
  constraint tangent L41 A41
  constraint tangent L42 A41
  constraint equal A41 A42
  constraint tangent L42 A43
  constraint tangent L43 A43
  constraint equal A42 A43
  constraint horizontal L44
  constraint vertical L45
  constraint horizontal L46
  constraint vertical L47
  constraint tangent L44 A46
  constraint tangent L47 A46
  constraint tangent L44 A44
  constraint tangent L45 A44
  constraint equal A44 A46
  constraint tangent L45 A45
  constraint tangent L46 A45
  constraint equal A45 A46
  constraint tangent L46 A47
  constraint tangent L47 A47
  constraint equal A46 A47
  constraint horizontal L48
  constraint vertical L49
  constraint horizontal L50
  constraint vertical L51
  constraint tangent L48 A50
  constraint tangent L51 A50
  constraint tangent L48 A48
  constraint tangent L49 A48
  constraint equal A48 A50
  constraint tangent L49 A49
  constraint tangent L50 A49
  constraint equal A49 A50
  constraint tangent L50 A51
  constraint tangent L51 A51
  constraint equal A50 A51
  constraint horizontal L52
  constraint vertical L53
  constraint horizontal L54
  constraint vertical L55
  constraint tangent L52 A54
  constraint tangent L55 A54
  constraint tangent L52 A52
  constraint tangent L53 A52
  constraint equal A52 A54
  constraint tangent L53 A53
  constraint tangent L54 A53
  constraint equal A53 A54
  constraint tangent L54 A55
  constraint tangent L55 A55
  constraint equal A54 A55
  constraint horizontal L56
  constraint vertical L57
  constraint horizontal L58
  constraint vertical L59
  constraint tangent L56 A58
  constraint tangent L59 A58
  constraint tangent L56 A56
  constraint tangent L57 A56
  constraint equal A56 A58
  constraint tangent L57 A57
  constraint tangent L58 A57
  constraint equal A57 A58
  constraint tangent L58 A59
  constraint tangent L59 A59
  constraint equal A58 A59
  constraint horizontal L60
  constraint vertical L61
  constraint horizontal L62
  constraint vertical L63
  constraint tangent L60 A62
  constraint tangent L63 A62
  constraint tangent L60 A60
  constraint tangent L61 A60
  constraint equal A60 A62
  constraint tangent L61 A61
  constraint tangent L62 A61
  constraint equal A61 A62
  constraint tangent L62 A63
  constraint tangent L63 A63
  constraint equal A62 A63
  constraint horizontal L64
  constraint vertical L65
  constraint horizontal L66
  constraint vertical L67
  constraint tangent L64 A66
  constraint tangent L67 A66
  constraint tangent L64 A64
  constraint tangent L65 A64
  constraint equal A64 A66
  constraint tangent L65 A65
  constraint tangent L66 A65
  constraint equal A65 A66
  constraint tangent L66 A67
  constraint tangent L67 A67
  constraint equal A66 A67
  constraint horizontal L68
  constraint vertical L69
  constraint horizontal L70
  constraint vertical L71
  constraint tangent L68 A70
  constraint tangent L71 A70
  constraint tangent L68 A68
  constraint tangent L69 A68
  constraint equal A68 A70
  constraint tangent L69 A69
  constraint tangent L70 A69
  constraint equal A69 A70
  constraint tangent L70 A71
  constraint tangent L71 A71
  constraint equal A70 A71
  constraint horizontal L72
  constraint vertical L73
  constraint horizontal L74
  constraint vertical L75
  constraint tangent L72 A74
  constraint tangent L75 A74
  constraint tangent L72 A72
  constraint tangent L73 A72
  constraint equal A72 A74
  constraint tangent L73 A73
  constraint tangent L74 A73
  constraint equal A73 A74
  constraint tangent L74 A75
  constraint tangent L75 A75
  constraint equal A74 A75
  constraint horizontal L76
  constraint vertical L77
  constraint horizontal L78
  constraint vertical L79
  constraint tangent L76 A78
  constraint tangent L79 A78
  constraint tangent L76 A76
  constraint tangent L77 A76
  constraint equal A76 A78
  constraint tangent L77 A77
  constraint tangent L78 A77
  constraint equal A77 A78
  constraint tangent L78 A79
  constraint tangent L79 A79
  constraint equal A78 A79
  constraint horizontal L80
  constraint vertical L81
  constraint horizontal L82
  constraint vertical L83
  constraint tangent L80 A82
  constraint tangent L83 A82
  constraint tangent L80 A80
  constraint tangent L81 A80
  constraint equal A80 A82
  constraint tangent L81 A81
  constraint tangent L82 A81
  constraint equal A81 A82
  constraint tangent L82 A83
  constraint tangent L83 A83
  constraint equal A82 A83
  constraint horizontal L84
  constraint vertical L85
  constraint horizontal L86
  constraint vertical L87
  constraint tangent L84 A86
  constraint tangent L87 A86
  constraint tangent L84 A84
  constraint tangent L85 A84
  constraint equal A84 A86
  constraint tangent L85 A85
  constraint tangent L86 A85
  constraint equal A85 A86
  constraint tangent L86 A87
  constraint tangent L87 A87
  constraint equal A86 A87
  constraint horizontal L88
  constraint vertical L89
  constraint horizontal L90
  constraint vertical L91
  constraint tangent L88 A90
  constraint tangent L91 A90
  constraint tangent L88 A88
  constraint tangent L89 A88
  constraint equal A88 A90
  constraint tangent L89 A89
  constraint tangent L90 A89
  constraint equal A89 A90
  constraint tangent L90 A91
  constraint tangent L91 A91
  constraint equal A90 A91
  constraint horizontal L92
  constraint vertical L93
  constraint horizontal L94
  constraint vertical L95
  constraint tangent L92 A94
  constraint tangent L95 A94
  constraint tangent L92 A92
  constraint tangent L93 A92
  constraint equal A92 A94
  constraint tangent L93 A93
  constraint tangent L94 A93
  constraint equal A93 A94
  constraint tangent L94 A95
  constraint tangent L95 A95
  constraint equal A94 A95
  constraint horizontal L96
  constraint vertical L97
  constraint horizontal L98
  constraint vertical L99
  constraint tangent L96 A98
  constraint tangent L99 A98
  constraint tangent L96 A96
  constraint tangent L97 A96
  constraint equal A96 A98
  constraint tangent L97 A97
  constraint tangent L98 A97
  constraint equal A97 A98
  constraint tangent L98 A99
  constraint tangent L99 A99
  constraint equal A98 A99
  constraint horizontal L100
  constraint vertical L101
  constraint horizontal L102
  constraint vertical L103
  constraint tangent L100 A102
  constraint tangent L103 A102
  constraint tangent L100 A100
  constraint tangent L101 A100
  constraint equal A100 A102
  constraint tangent L101 A101
  constraint tangent L102 A101
  constraint equal A101 A102
  constraint tangent L102 A103
  constraint tangent L103 A103
  constraint equal A102 A103
  constraint horizontal L104
  constraint vertical L105
  constraint horizontal L106
  constraint vertical L107
  constraint tangent L104 A106
  constraint tangent L107 A106
  constraint tangent L104 A104
  constraint tangent L105 A104
  constraint equal A104 A106
  constraint tangent L105 A105
  constraint tangent L106 A105
  constraint equal A105 A106
  constraint tangent L106 A107
  constraint tangent L107 A107
  constraint equal A106 A107
  constraint horizontal L108
  constraint vertical L109
  constraint horizontal L110
  constraint vertical L111
  constraint tangent L108 A110
  constraint tangent L111 A110
  constraint tangent L108 A108
  constraint tangent L109 A108
  constraint equal A108 A110
  constraint tangent L109 A109
  constraint tangent L110 A109
  constraint equal A109 A110
  constraint tangent L110 A111
  constraint tangent L111 A111
  constraint equal A110 A111
  constraint horizontal L112
  constraint vertical L113
  constraint horizontal L114
  constraint vertical L115
  constraint tangent L112 A114
  constraint tangent L115 A114
  constraint tangent L112 A112
  constraint tangent L113 A112
  constraint equal A112 A114
  constraint tangent L113 A113
  constraint tangent L114 A113
  constraint equal A113 A114
  constraint tangent L114 A115
  constraint tangent L115 A115
  constraint equal A114 A115
  constraint horizontal L116
  constraint vertical L117
  constraint horizontal L118
  constraint vertical L119
  constraint tangent L116 A118
  constraint tangent L119 A118
  constraint tangent L116 A116
  constraint tangent L117 A116
  constraint equal A116 A118
  constraint tangent L117 A117
  constraint tangent L118 A117
  constraint equal A117 A118
  constraint tangent L118 A119
  constraint tangent L119 A119
  constraint equal A118 A119
  constraint horizontal L120
  constraint vertical L121
  constraint horizontal L122
  constraint vertical L123
  constraint tangent L120 A122
  constraint tangent L123 A122
  constraint tangent L120 A120
  constraint tangent L121 A120
  constraint equal A120 A122
  constraint tangent L121 A121
  constraint tangent L122 A121
  constraint equal A121 A122
  constraint tangent L122 A123
  constraint tangent L123 A123
  constraint equal A122 A123
  constraint horizontal L124
  constraint vertical L125
  constraint horizontal L126
  constraint vertical L127
  constraint tangent L124 A126
  constraint tangent L127 A126
  constraint tangent L124 A124
  constraint tangent L125 A124
  constraint equal A124 A126
  constraint tangent L125 A125
  constraint tangent L126 A125
  constraint equal A125 A126
  constraint tangent L126 A127
  constraint tangent L127 A127
  constraint equal A126 A127
  constraint horizontal L128
  constraint vertical L129
  constraint horizontal L130
  constraint vertical L131
  constraint tangent L128 A130
  constraint tangent L131 A130
  constraint tangent L128 A128
  constraint tangent L129 A128
  constraint equal A128 A130
  constraint tangent L129 A129
  constraint tangent L130 A129
  constraint equal A129 A130
  constraint tangent L130 A131
  constraint tangent L131 A131
  constraint equal A130 A131
  constraint horizontal L132
  constraint vertical L133
  constraint horizontal L134
  constraint vertical L135
  constraint tangent L132 A134
  constraint tangent L135 A134
  constraint tangent L132 A132
  constraint tangent L133 A132
  constraint equal A132 A134
  constraint tangent L133 A133
  constraint tangent L134 A133
  constraint equal A133 A134
  constraint tangent L134 A135
  constraint tangent L135 A135
  constraint equal A134 A135
  constraint horizontal L136
  constraint vertical L137
  constraint horizontal L138
  constraint vertical L139
  constraint tangent L136 A138
  constraint tangent L139 A138
  constraint tangent L136 A136
  constraint tangent L137 A136
  constraint equal A136 A138
  constraint tangent L137 A137
  constraint tangent L138 A137
  constraint equal A137 A138
  constraint tangent L138 A139
  constraint tangent L139 A139
  constraint equal A138 A139
  constraint horizontal L140
  constraint vertical L141
  constraint horizontal L142
  constraint vertical L143
  constraint tangent L140 A142
  constraint tangent L143 A142
  constraint tangent L140 A140
  constraint tangent L141 A140
  constraint equal A140 A142
  constraint tangent L141 A141
  constraint tangent L142 A141
  constraint equal A141 A142
  constraint tangent L142 A143
  constraint tangent L143 A143
  constraint equal A142 A143
  constraint horizontal L144
  constraint vertical L145
  constraint horizontal L146
  constraint vertical L147
  constraint tangent L144 A146
  constraint tangent L147 A146
  constraint tangent L144 A144
  constraint tangent L145 A144
  constraint equal A144 A146
  constraint tangent L145 A145
  constraint tangent L146 A145
  constraint equal A145 A146
  constraint tangent L146 A147
  constraint tangent L147 A147
  constraint equal A146 A147
  constraint horizontal L148
  constraint vertical L149
  constraint horizontal L150
  constraint vertical L151
  constraint tangent L148 A150
  constraint tangent L151 A150
  constraint tangent L148 A148
  constraint tangent L149 A148
  constraint equal A148 A150
  constraint tangent L149 A149
  constraint tangent L150 A149
  constraint equal A149 A150
  constraint tangent L150 A151
  constraint tangent L151 A151
  constraint equal A150 A151
  constraint horizontal L152
  constraint vertical L153
  constraint horizontal L154
  constraint vertical L155
  constraint tangent L152 A154
  constraint tangent L155 A154
  constraint tangent L152 A152
  constraint tangent L153 A152
  constraint equal A152 A154
  constraint tangent L153 A153
  constraint tangent L154 A153
  constraint equal A153 A154
  constraint tangent L154 A155
  constraint tangent L155 A155
  constraint equal A154 A155
  constraint horizontal L156
  constraint vertical L157
  constraint horizontal L158
  constraint vertical L159
  constraint tangent L156 A158
  constraint tangent L159 A158
  constraint tangent L156 A156
  constraint tangent L157 A156
  constraint equal A156 A158
  constraint tangent L157 A157
  constraint tangent L158 A157
  constraint equal A157 A158
  constraint tangent L158 A159
  constraint tangent L159 A159
  constraint equal A158 A159
  constraint horizontal L160
  constraint vertical L161
  constraint horizontal L162
  constraint vertical L163
  constraint tangent L160 A162
  constraint tangent L163 A162
  constraint tangent L160 A160
  constraint tangent L161 A160
  constraint equal A160 A162
  constraint tangent L161 A161
  constraint tangent L162 A161
  constraint equal A161 A162
  constraint tangent L162 A163
  constraint tangent L163 A163
  constraint equal A162 A163
  constraint horizontal L164
  constraint vertical L165
  constraint horizontal L166
  constraint vertical L167
  constraint tangent L164 A166
  constraint tangent L167 A166
  constraint tangent L164 A164
  constraint tangent L165 A164
  constraint equal A164 A166
  constraint tangent L165 A165
  constraint tangent L166 A165
  constraint equal A165 A166
  constraint tangent L166 A167
  constraint tangent L167 A167
  constraint equal A166 A167
  constraint horizontal L168
  constraint vertical L169
  constraint horizontal L170
  constraint vertical L171
  constraint tangent L168 A170
  constraint tangent L171 A170
  constraint tangent L168 A168
  constraint tangent L169 A168
  constraint equal A168 A170
  constraint tangent L169 A169
  constraint tangent L170 A169
  constraint equal A169 A170
  constraint tangent L170 A171
  constraint tangent L171 A171
  constraint equal A170 A171
  constraint horizontal L172
  constraint vertical L173
  constraint horizontal L174
  constraint vertical L175
  constraint tangent L172 A174
  constraint tangent L175 A174
  constraint tangent L172 A172
  constraint tangent L173 A172
  constraint equal A172 A174
  constraint tangent L173 A173
  constraint tangent L174 A173
  constraint equal A173 A174
  constraint tangent L174 A175
  constraint tangent L175 A175
  constraint equal A174 A175
  constraint horizontal L176
  constraint vertical L177
  constraint horizontal L178
  constraint vertical L179
  constraint tangent L176 A178
  constraint tangent L179 A178
  constraint tangent L176 A176
  constraint tangent L177 A176
  constraint equal A176 A178
  constraint tangent L177 A177
  constraint tangent L178 A177
  constraint equal A177 A178
  constraint tangent L178 A179
  constraint tangent L179 A179
  constraint equal A178 A179
  constraint horizontal L180
  constraint vertical L181
  constraint horizontal L182
  constraint vertical L183
  constraint tangent L180 A182
  constraint tangent L183 A182
  constraint tangent L180 A180
  constraint tangent L181 A180
  constraint equal A180 A182
  constraint tangent L181 A181
  constraint tangent L182 A181
  constraint equal A181 A182
  constraint tangent L182 A183
  constraint tangent L183 A183
  constraint equal A182 A183
  constraint horizontal L184
  constraint vertical L185
  constraint horizontal L186
  constraint vertical L187
  constraint tangent L184 A186
  constraint tangent L187 A186
  constraint tangent L184 A184
  constraint tangent L185 A184
  constraint equal A184 A186